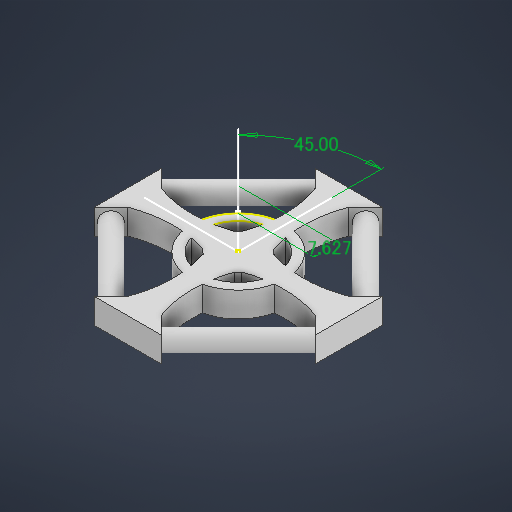
# Autodesk Inventor part: Part2
Saved by Autodesk Inventor 2026 (Build 300175000, 175)
## iProperties
Created: 2025-10-15
Part Number: Part2
Material: 一般
Document SubType Name: Modeling
Designer: masak
Density: 1 g/cm^3
Appearance: 既定
Author: masak
Autodesk Inventor part; units mm, degrees
ref_plane "YZ Plane" through (0, 0, 0) normal (1, 0, 0) x (0, 1, 0)
ref_plane "XZ Plane" through (0, 0, 0) normal (0, 1, 0) x (-1, 0, 0)
ref_plane "XY Plane" through (0, 0, 0) normal (0, 0, 1) x (1, 0, 0)
sketch "スケッチ1" plane through (0, 0, 0) normal (0, 1, 0) x (-1, 0, 0)
  line L0 (-35.3553, 0) -> (0, 35.3553)
  line L1 (0, 35.3553) -> (35.3553, 0)
  line L2 (35.3553, 0) -> (0, -35.3553)
  line L3 (0, -35.3553) -> (-35.3553, 0)
  line L4 (-25, 25) -> (25, -25) construction
  line L5 (25, 25) -> (-25, -25) construction
  line L6 (0, 0) -> (0, -30)
  line L7 (0, -30) -> (5.3553, -30)
  line L8 (5.3553, -30) -> (10.7107, -35.3553)
  line L9 (5.3553, -30) -> (5.3553, 0)
  line L10 (0, 0) -> (30, 0)
  line L11 (30, 0) -> (30, -5.3553)
  line L12 (30, -5.3553) -> (0, -5.3553)
  line L13 (35.3553, 0) -> (47.1243, -11.769)
  line L14 (35.3553, 0) -> (35.3553, -35.3553)
  line L15 (0, -35.3553) -> (35.3553, -35.3553)
  line L16 (30, -5.3553) -> (35.3553, -10.7107)
  line L17 (5.3553, 30) -> (5.3553, 0)
  line L18 (30, 5.3553) -> (0, 5.3553)
  line L19 (0, 35.3553) -> (35.3553, 0)
  line L20 (30, 5.3553) -> (35.3553, 10.7107)
  line L21 (30, 0) -> (30, 5.3553)
  line L22 (0, 30) -> (5.3553, 30)
  line L23 (5.3553, 30) -> (10.7107, 35.3553)
  line L24 (0, 35.3553) -> (35.3553, 35.3553)
  line L25 (35.3553, 0) -> (35.3553, 35.3553)
  line L26 (0, 0) -> (0, 30)
  line L27 (0, 0) -> (30, 0)
  line L28 (-30, 5.3553) -> (0, 5.3553)
  line L29 (-5.3553, 30) -> (-5.3553, 0)
  line L30 (-35.3553, 0) -> (0, 35.3553)
  line L31 (-5.3553, 30) -> (-10.7107, 35.3553)
  line L32 (0, 30) -> (-5.3553, 30)
  line L33 (-30, 0) -> (-30, 5.3553)
  line L34 (-30, 5.3553) -> (-35.3553, 10.7107)
  line L35 (-35.3553, 0) -> (-35.3553, 35.3553)
  line L36 (0, 35.3553) -> (-35.3553, 35.3553)
  line L37 (0, 0) -> (-30, 0)
  line L38 (0, 0) -> (0, 30)
  line L39 (-5.3553, -30) -> (-5.3553, 0)
  line L40 (-30, -5.3553) -> (0, -5.3553)
  line L41 (0, -35.3553) -> (-35.3553, 0)
  line L42 (-30, -5.3553) -> (-35.3553, -10.7107)
  line L43 (-30, 0) -> (-30, -5.3553)
  line L44 (0, -30) -> (-5.3553, -30)
  line L45 (-5.3553, -30) -> (-10.7107, -35.3553)
  line L46 (0, -35.3553) -> (-35.3553, -35.3553)
  line L47 (-35.3553, 0) -> (-35.3553, -35.3553)
  line L48 (0, 0) -> (0, -30)
  line L49 (0, 0) -> (-30, 0)
  point P0 (35.3553, 0)
  point P1 (5.3553, 5.3553)
  point P2 (-5.3553, 5.3553)
  point P3 (-5.3553, -5.3553)
  point P4 (0, -35.3553)
  point P5 (5.3553, -5.3553)
  dimension "d0" = 50
  dimension "d1" = 50
  dimension "d3" = 30
  dimension "d4" = 30
  dimension "d7" = 360
  constraints: 100 end point, 16 point on line, 4 vertical, 3 perpendicular, 2 coincident, 2 horizontal, 2 midpoint, 2 parallel, 95 other
  measures "d0" distance of L0.end L1.end
  measures "d1" distance of L1.end L2.end
  measures "d3" distance of L6.start L6.end
  measures "d4" distance of L6.start L10.end
extrude "押し出し1" add sketch "スケッチ1" along normal mid plane 8 contours L35 L34 L0 | L0 L33 L43 L3 | L3 L42 L47 | L28 L29 L37 L33 | L43 L37 L39 L40 | L31 L36 L0 | L32 L26 L28 L29 | L0 L1 L22 L32 | L28 L26 L37 L29 | L44 L7 L2 L3 | L39 L40 L6 L44 | L3 L46 L45 | L39 L37 L6 L40 | L24 L23 L1 | L22 L17 L18 L26 | L18 L17 L10 L26 | L2 L8 L15 | L6 L12 L9 L7 | L6 L10 L9 L12 | L18 L21 L10 L17 | L9 L10 L11 L12 | L20 L25 L1 | L1 L2 L11 L21 | L2 L14 L16
sketch "スケッチ3" plane through (5.3553, -4, 30) normal (0.7071068, 0, -0.7071068) x (-0.7071068, 0, -0.7071068)
  line L0 (-7.5736, 8) -> (7.5736, 8) projected
  line L1 (17.4264, 0) -> (0, 0) projected
  line L2 (-7.5736, 8) -> (0, 0)
  line L3 (-7.5736, 0) -> (7.5736, 0) projected
  line L4 (0, 8) -> (-7.5736, 0)
  circle A0 centre (-3.7868, 4) radius 3
  point P0 (25, 4)
  dimension "d12" = 6
  constraints: 4 end point, 2 midpoint, 1 centre point, 1 coincident
  measures "d12" diameter of A0
extrude "押し出し2" add sketch "スケッチ3" along normal blind 35 contours A0 L4 L2 | L2 L4 A0 | A0 L2 L4 | L2 A0 L4
pattern_circular "円形状パターン1" count 4 over 360 about axis through (0, -10, 0) along (0, 1, 0) of "押し出し2"
sketch "スケッチ4" plane through (0, 4, 0) normal (0, 1, 0) x (1, 0, 0)
  line L0 (-30, -5.3553) -> (-5.3553, -5.3553) projected
  line L1 (-35.3553, -10.7107) -> (-30, -5.3553) projected
  arc A0 (-5.3553, -5.3553) -> (-30, -5.3553) centre (-17.6777, -37.7141) ccw
  line L2 (-30, -5.3553) -> (-5.3553, -5.3553)
  line L3 (-35.3553, 0) -> (35.3553, 0)
  line L4 (35.3553, -10.7107) -> (35.3553, 10.7107) projected
  line L5 (10.7107, 35.3553) -> (-10.7107, 35.3553) projected
  line L6 (0, 35.3553) -> (0, -35.3553)
  arc A1 (-30, 5.3553) -> (-5.3553, 5.3553) centre (-17.6777, 37.7141) ccw
  arc A2 (5.3553, -5.3553) -> (5.3553, -30) centre (37.7141, -17.6777) ccw
  line L7 (5.3553, -30) -> (5.3553, -5.3553)
  arc A3 (-5.3553, -30) -> (-5.3553, -5.3553) centre (-37.7141, -17.6777) ccw
  arc A4 (5.3553, 5.3553) -> (30, 5.3553) centre (17.6777, 37.7141) ccw
  line L8 (30, 5.3553) -> (5.3553, 5.3553)
  arc A5 (30, -5.3553) -> (5.3553, -5.3553) centre (17.6777, -37.7141) ccw
  arc A6 (-5.3553, 5.3553) -> (-5.3553, 30) centre (-37.7141, 17.6777) ccw
  line L9 (-5.3553, 30) -> (-5.3553, 5.3553)
  arc A7 (5.3553, 30) -> (5.3553, 5.3553) centre (37.7141, 17.6777) ccw
  line L10 (-30, 5.3553) -> (-35.3553, 10.7107) projected
  line L11 (-30, 5.3553) -> (-5.3553, 5.3553) projected
  line L12 (-30, 5.3553) -> (-5.3553, 5.3553)
  line L13 (-5.3553, 30) -> (-5.3553, 5.3553)
  line L14 (5.3553, 30) -> (5.3553, 5.3553)
  line L15 (5.3553, -5.3553) -> (30, -5.3553)
  line L16 (10.7107, -35.3553) -> (5.3553, -30) projected
  line L17 (5.3553, -5.3553) -> (5.3553, -30)
  line L18 (-5.3553, -5.3553) -> (-5.3553, -30)
  point P0 (0, 0)
  point P1 (-5.3553, 5.3553)
  point P2 (-5.3553, 5.3553)
  point P3 (5.3553, 5.3553)
  point P4 (5.3553, 5.3553)
  point P5 (5.3553, 5.3553)
  point P6 (5.3553, 5.3553)
  dimension "d20" = 360
  constraints: 24 end point, 17 point on circle, 8 centre point, 4 vertical, 3 symmetric about line, 2 midpoint, 1 collinear, 1 horizontal, 1 perpendicular, 38 other
extrude "押し出し3" cut sketch "スケッチ4" against normal blind 8
sketch "スケッチ5" plane through (0, 4, 0) normal (0, 1, 0) x (1, 0, 0)
  circle A0 centre (0, 0) radius 15
  circle A1 centre (0, 0) radius 12
  circle A2 centre (0, 0) radius 8
  circle A3 centre (0, 0) radius 3
  dimension "d24" = 30
  dimension "d25" = 6
  dimension "d26" = 24
  dimension "d27" = 16
  constraints: 4 centre point, 4 coincident
  measures "d24" diameter of A0
  measures "d25" diameter of A3
  measures "d26" diameter of A1
  measures "d27" diameter of A2
extrude "押し出し4" add sketch "スケッチ5" against normal blind 8 contours A0 | A2 | A3
sketch "スケッチ6" plane through (0, 4, 0) normal (0, 1, 0) x (1, 0, 0)
  line L0 (0, 0) -> (0, 29.8469)
  line L1 (0, 0) -> (-29.8987, 0)
  line L2 (0, 0) -> (-33.9676, 33.9676)
  arc A0 (-3.657, 11.4292) -> (-11.4292, 3.657) centre (0, 0) ccw projected
  line L3 (0, 0) -> (-18.2338, 18.2338)
  line L4 (0, 0) -> (-10.6189, 10.6189)
  line L5 (-18.2338, 18.2338) -> (-10.6189, 10.6189)
  arc A1 (-3.2212, 14.6501) -> (-14.6501, 3.2212) centre (0, 0) ccw projected
  point P0 (-10.6066, 10.6066)
  dimension "d30" = 45
  dimension "d31" = 7.6272
  constraints: 12 end point, 2 point on line, 1 collinear, 1 horizontal, 1 point on circle, 1 vertical
  measures "d30" angle of L0 L2
  measures "d31" horizontal distance of point (-10.607, 10.607) L3.end
